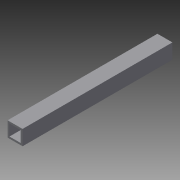
# Autodesk Inventor part: Part3
Saved by Autodesk Inventor 2015 (Build 190159000, 159)
## iProperties
Created: 2015-07-04
Part Number: Part3
Material: Generic
Document SubType Name: Modeling
Designer: tsayman
Density: 1 g/cm^3
Appearance: Default
Author: tsayman
Autodesk Inventor part; units mm, degrees
ref_plane "YZ Plane" through (0, 0, 0) normal (1, 0, 0) x (0, 1, 0)
ref_plane "XZ Plane" through (0, 0, 0) normal (0, 1, 0) x (-1, 0, 0)
ref_plane "XY Plane" through (0, 0, 0) normal (0, 0, 1) x (1, 0, 0)
sketch "Sketch1" plane through (0, 0, 0) normal (0, 1, 0) x (-1, 0, 0)
  line L0 (-34.4448, -75.6525) -> (-9.0448, -75.6525)
  line L1 (-9.0448, -75.6525) -> (-9.0448, -329.6525)
  line L2 (-9.0448, -329.6525) -> (-34.4448, -329.6525)
  line L3 (-34.4448, -329.6525) -> (-34.4448, -75.6525)
  point P0 (0, 0)
  dimension "d0" = 25.4
  dimension "d1" = 254
  constraints: 8 end point, 2 parallel, 1 horizontal, 1 perpendicular
  measures "d0" distance of L1.end L2.end
  measures "d1" distance of L0.end L1.end
extrude "Extrusion1" add sketch "Sketch1" along normal blind 25.4
shell "Shell1" thickness 3.175 removed faces 2 at (25.9782, 8.4667, -75.6525) at (17.5115, 16.9333, -329.6525)
body "Solid1"
